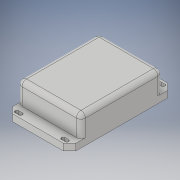
# Autodesk Inventor part: 24v Converter
Saved by Autodesk Inventor 2017 (Build 210142000, 142)
## iProperties
Created: 2017-02-10
Part Number: 24v Converter
Material: Generic
Document SubType Name: Modeling
Designer: michael
Density: 1 g/cm^3
Appearance: Default
Author: michael
Autodesk Inventor part; units mm, degrees
ref_plane "YZ Plane" through (0, 0, 0) normal (1, 0, 0) x (0, 1, 0)
ref_plane "XZ Plane" through (0, 0, 0) normal (0, 1, 0) x (-1, 0, 0)
ref_plane "XY Plane" through (0, 0, 0) normal (0, 0, 1) x (1, 0, 0)
sketch "Sketch1" plane through (0, 0, 0) normal (0, 1, 0) x (-1, 0, 0)
  line L0 (-44.45, 73.025) -> (44.45, 73.025)
  line L1 (44.45, 73.025) -> (44.45, -73.025)
  line L2 (44.45, -73.025) -> (-44.45, -73.025)
  line L3 (-44.45, -73.025) -> (-44.45, 73.025)
  line L4 (-44.45, 73.025) -> (44.45, -73.025) construction
  line L5 (44.45, 73.025) -> (-44.45, -73.025) construction
  point P0 (0, 0)
  dimension "d0" = 88.9
  dimension "d1" = 146.05
  constraints: 12 end point, 2 midpoint, 2 parallel, 1 horizontal, 1 perpendicular
  measures "d0" distance of L1.end L2.end
  measures "d1" distance of L0.end L1.end
extrude "Extrusion1" add sketch "Sketch1" along normal blind 9.525
sketch "Sketch2" plane through (0, 9.525, 0) normal (0, 1, 0) x (1, 0, 0)
  line L0 (44.45, -57.15) -> (-44.45, -57.15)
  line L1 (-44.45, -57.15) -> (-44.45, 57.15)
  line L2 (-44.45, 57.15) -> (44.45, 57.15)
  line L3 (44.45, 57.15) -> (44.45, -57.15)
  line L4 (44.45, -57.15) -> (-44.45, 57.15) construction
  line L5 (-44.45, -57.15) -> (44.45, 57.15) construction
  point P0 (0, 0)
  dimension "d4" = 88.9
  dimension "d5" = 114.3
  constraints: 12 end point, 2 midpoint, 2 parallel, 1 horizontal, 1 perpendicular
  measures "d4" distance of L1.end L2.end
  measures "d5" distance of L0.end L1.end
extrude "Extrusion2" add sketch "Sketch2" along normal blind 30
sketch "Sketch3" plane through (0, 0, 0) normal (0, -1, 0) x (1, 0, 0)
  line L0 (-37.5007, -70.0145) -> (-27.5007, -70.0145)
  line L1 (-27.5007, -70.0145) -> (-27.5007, -65.0145)
  line L2 (-27.5007, -65.0145) -> (-37.5007, -65.0145)
  line L3 (-37.5007, -65.0145) -> (-37.5007, -70.0145)
  line L4 (-37.5007, -70.0145) -> (-27.5007, -65.0145) construction
  line L5 (-27.5007, -70.0145) -> (-37.5007, -65.0145) construction
  line L6 (-37.5007, 64.9855) -> (-27.5007, 64.9855)
  line L7 (-27.5007, 64.9855) -> (-27.5007, 69.9855)
  line L8 (-27.5007, 69.9855) -> (-37.5007, 69.9855)
  line L9 (-37.5007, 69.9855) -> (-37.5007, 64.9855)
  line L10 (-37.5007, 64.9855) -> (-27.5007, 69.9855) construction
  line L11 (-27.5007, 64.9855) -> (-37.5007, 69.9855) construction
  line L12 (-44.45, -73.025) -> (44.45, -73.025) projected
  line L13 (27.4993, -70.0145) -> (37.4993, -70.0145)
  line L14 (37.4993, -70.0145) -> (37.4993, -65.0145)
  line L15 (37.4993, -65.0145) -> (27.4993, -65.0145)
  line L16 (27.4993, -65.0145) -> (27.4993, -70.0145)
  line L17 (27.4993, -70.0145) -> (37.4993, -65.0145) construction
  line L18 (37.4993, -70.0145) -> (27.4993, -65.0145) construction
  line L19 (44.45, -73.025) -> (44.45, 73.025) projected
  line L20 (37.4993, 69.9855) -> (27.4993, 69.9855)
  line L21 (27.4993, 69.9855) -> (27.4993, 64.9855)
  line L22 (27.4993, 64.9855) -> (37.4993, 64.9855)
  line L23 (37.4993, 64.9855) -> (37.4993, 69.9855)
  line L24 (37.4993, 69.9855) -> (27.4993, 64.9855) construction
  line L25 (27.4993, 69.9855) -> (37.4993, 64.9855) construction
  point P0 (0, 0)
  point P1 (-32.5007, -67.5145)
  point P2 (-32.5007, 67.4855)
  point P3 (32.4993, -67.5145)
  point P4 (-42.8625, -71.4375)
  point P5 (32.4993, 67.4855)
  dimension "d8" = 10
  dimension "d9" = 5
  dimension "d10" = 10
  dimension "d11" = 5
  dimension "d12" = 0
  dimension "d13" = 135
  dimension "d14" = 5.5105
  dimension "d15" = 10
  dimension "d16" = 5
  dimension "d17" = 65
  dimension "d18" = 5.5105
  dimension "d19" = 11.9507
  dimension "d20" = 5
  dimension "d21" = 10
  dimension "d22" = 135
  dimension "d23" = 11.9507
  constraints: 48 end point, 8 midpoint, 8 parallel, 4 horizontal, 4 perpendicular
  measures "d8" distance of L2.end L1.end
  measures "d9" distance of L1.end L0.end
  measures "d10" distance of L8.end L7.end
  measures "d11" distance of L7.end L6.end
  measures "d12" horizontal distance of point (-32.501, 67.486) point (-32.501, -67.514)
  measures "d13" distance of point (-32.501, -67.514) point (-32.501, 67.486)
  measures "d14" distance from line of L12 point (-32.501, -67.514)
  measures "d15" distance of L15.end L14.end
  measures "d16" distance of L14.end L13.end
  measures "d17" distance of point (-32.501, -67.514) point (32.499, -67.514)
  measures "d18" distance from line of L12 point (32.499, -67.514)
  measures "d19" distance from line of L19 point (32.499, -67.514)
  measures "d20" distance between parallel lines of L20 L22
  measures "d21" distance between parallel lines of L23 L21
  measures "d22" distance of point (32.499, -67.514) point (32.499, 67.486)
  measures "d23" distance from line of L19 point (32.499, 67.486)
extrude "Extrusion3" cut sketch "Sketch3" against normal blind 30
fillet "Fillet1" radius 2.159 16 edges at (-27.5007, 4.7625, 64.9855) (-27.5007, 4.7625, 69.9855) (-37.5007, 4.7625, 69.9855) (-37.5007, 4.7625, 64.9855) (37.4993, 4.7625, 64.9855) (37.4993, 4.7625, 69.9855) (27.4993, 4.7625, 64.9855) (27.4993, 4.7625, 69.9855) (27.4993, 4.7625, -65.0145) (37.4993, 4.7625, -70.0145) (37.4993, 4.7625, -65.0145) (27.4993, 4.7625, -70.0145) (-27.5007, 4.7625, -65.0145) (-27.5007, 4.7625, -70.0145) (-37.5007, 4.7625, -65.0145) (-37.5007, 4.7625, -70.0145)
fillet "Fillet2" radius 6.35 1 edges at (-44.45, 24.525, -57.15)
fillet "Fillet3" radius 6.35 8 edges at (-44.45, 24.525, 57.15) (44.45, 24.525, 57.15) (44.45, 24.525, -57.15) (-42.5901, 39.525, -55.2901) (-44.45, 39.525, 3.175) (3.175, 39.525, -57.15) (44.45, 39.525, 0) (0, 39.525, 57.15)
chamfer "Chamfer1" distance 8.89 angle 45 4 edges at (44.45, 4.7625, 73.025) (-44.45, 4.7625, 73.025) (44.45, 4.7625, -73.025) (-44.45, 4.7625, -73.025)
equation "\"d18\" = d14"
equation "\"d20\" = d11"
equation "\"d21\" = d10"
equation "\"d22\" = d13"
equation "\"d23\" = d19"
body "Solid1"
